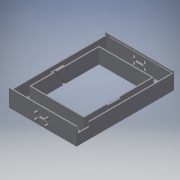
# Autodesk Inventor part: Frame V2.3
Saved by Autodesk Inventor 2018.3 (Build 223284000, 284)
## iProperties
Created: 2020-11-27
Part Number: Frame V2.3
Material: Generic
Document SubType Name: Modeling
Designer: daanv
Density: 1 g/cm^3
Appearance: Default
Author: daanv
Autodesk Inventor part; units mm, degrees
ref_plane "YZ Plane" through (0, 0, 0) normal (1, 0, 0) x (0, 1, 0)
ref_plane "XZ Plane" through (0, 0, 0) normal (0, 1, 0) x (-1, 0, 0)
ref_plane "XY Plane" through (0, 0, 0) normal (0, 0, 1) x (1, 0, 0)
sketch "Sketch1" plane through (0, 0, 0) normal (0, 0, 1) x (1, 0, 0)
  line L0 (0, 0) -> (90, 0)
  line L1 (90, 0) -> (90, 130)
  line L2 (90, 130) -> (0, 130)
  line L3 (0, 130) -> (0, 0)
  line L4 (10, 20) -> (80, 20)
  line L5 (80, 20) -> (80, 110)
  line L6 (80, 110) -> (10, 110)
  line L7 (10, 110) -> (10, 20)
  dimension "d0" = 90
  dimension "d1" = 130
  dimension "d2" = 70
  dimension "d3" = 90
  dimension "d16" = 20
  dimension "d17" = 20
  dimension "d18" = 10
  constraints: 16 end point, 4 parallel, 2 horizontal, 2 perpendicular
  measures "d0" distance of L2.end L1.end
  measures "d1" distance of L1.end L0.end
  measures "d2" distance of L6.end L5.end
  measures "d3" distance of L5.end L4.end
  measures "d16" distance between parallel lines of L2 L6
  measures "d17" distance between parallel lines of L0 L4
  measures "d18" distance between parallel lines of L1 L5
extrude "Extrusion1" add sketch "Sketch1" along normal blind 20
sketch "Sketch2" plane through (10, 20, 0) normal (1, 0, 0) x (0, 0, -1)
  line L0 (0, 90) -> (0, 0) projected
  line L1 (0, 42.1132) -> (-20, 30.5662)
  line L2 (-20, 110) -> (-20, -20) projected
  line L3 (0, 42.1132) -> (23.094, 42.1132) construction
  line L4 (-20, 30.5662) -> (-20, 33.6662)
  line L5 (-20, 33.6662) -> (0, 45.2132)
  line L6 (0, 42.1132) -> (0, 45.2132)
  point P0 (-20, 0)
  point P1 (0, -20)
  dimension "d6" = 210
  dimension "d7" = 3.1
  dimension "d8" = 26.4711
  constraints: 10 end point, 4 point on line, 1 collinear, 1 equal length, 1 horizontal, 1 parallel
  measures "d7" distance of L1.end L4.end
  measures "d8" distance from line of point (-20, 0) L1
extrude "Extrusion2" cut sketch "Sketch2" against normal blind 2.1
sketch "Sketch3" plane through (80, 20, 0) normal (-1, 0, 0) x (0, 0, 1)
  line L0 (0, 0) -> (0, 90) projected
  line L1 (20, 90) -> (20, 0) projected
  line L2 (0, 42.1132) -> (20, 30.5662)
  line L3 (0, 42.1132) -> (23.094, 42.1132) construction
  line L4 (20, 30.5662) -> (20, 33.6662)
  line L5 (20, 33.6662) -> (0, 45.2132)
  line L6 (0, 42.1132) -> (0, 45.2132)
  point P0 (0, -20)
  dimension "d11" = 30
  dimension "d12" = 3.1
  dimension "d13" = 26.4711
  constraints: 10 end point, 4 point on line, 1 equal length, 1 horizontal, 1 parallel
  measures "d11" angle of L2 L3
  measures "d12" distance of L2.end L4.end
  measures "d13" distance from line of L1.end L2
extrude "Extrusion3" cut sketch "Sketch3" against normal blind 2.1
sketch "Sketch4" plane through (0, 0, 0) normal (0, -1, 0) x (1, 0, 0)
  line L0 (0, 0) -> (90, 0) projected
  line L1 (90, 0) -> (90, 20) projected
  line L2 (0, 20) -> (90, 20) projected
  line L3 (0, 0) -> (0, 20) projected
  line L4 (55, 3) -> (35, 3)
  line L5 (35, 3) -> (35, 17)
  line L6 (35, 17) -> (55, 17)
  line L7 (55, 17) -> (55, 3)
  line L8 (53.2053, 7.41) -> (53.87, 5.3643)
  line L9 (53.87, 5.3643) -> (52.1298, 4.1)
  line L10 (52.1298, 4.1) -> (50.3897, 5.3643)
  line L11 (50.3897, 5.3643) -> (51.0543, 7.41)
  line L12 (51.0543, 7.41) -> (53.2053, 7.41)
  line L13 (38.9443, 7.41) -> (39.609, 5.3643)
  line L14 (39.609, 5.3643) -> (37.8689, 4.1)
  line L15 (37.8689, 4.1) -> (36.1287, 5.3643)
  line L16 (36.1287, 5.3643) -> (36.7934, 7.41)
  line L17 (36.7934, 7.41) -> (38.9443, 7.41)
  line L18 (38.9447, 15.55) -> (39.6093, 13.5043)
  line L19 (39.6093, 13.5043) -> (37.8692, 12.24)
  line L20 (37.8692, 12.24) -> (36.129, 13.5043)
  line L21 (36.129, 13.5043) -> (36.7937, 15.55)
  line L22 (36.7937, 15.55) -> (38.9447, 15.55)
  line L23 (53.2053, 15.55) -> (53.87, 13.5043)
  line L24 (53.87, 13.5043) -> (52.1298, 12.24)
  line L25 (52.1298, 12.24) -> (50.3897, 13.5043)
  line L26 (50.3897, 13.5043) -> (51.0543, 15.55)
  line L27 (51.0543, 15.55) -> (53.2053, 15.55)
  point P0 (52.1298, 5.9297)
  point P1 (37.8689, 5.9297)
  point P2 (37.8692, 14.0697)
  point P3 (52.1298, 14.0697)
  dimension "d19" = 20
  dimension "d20" = 14
  dimension "d21" = 3
  dimension "d22" = 3
  dimension "d23" = 35
  dimension "d24" = 35
  dimension "d25" = 1.45
  dimension "d26" = 1.45
  dimension "d27" = 1.1
  dimension "d28" = 1.1
  dimension "d29" = 12.11
  dimension "d30" = 1.13
  dimension "d31" = 1.13
  dimension "d32" = 4.83
  dimension "d33" = 4.83
  dimension "d34" = 1.129
  dimension "d35" = 1.1287
  constraints: 48 end point, 5 horizontal, 3 equal length, 2 parallel, 1 perpendicular, 44 other
  measures "d19" distance of L5.end L6.end
  measures "d20" distance of L4.end L5.end
  measures "d21" distance between parallel lines of L4 L0
  measures "d22" distance between parallel lines of L2 L6
  measures "d23" distance between parallel lines of L1 L7
  measures "d24" distance between parallel lines of L3 L5
  measures "d25" distance between parallel lines of L6 L27
  measures "d26" distance between parallel lines of L22 L6
  measures "d27" distance from line of L4 L9.end
  measures "d28" distance from line of L4 L14.end
  measures "d29" distance of L13.start L11.end
  measures "d30" distance from line of L7 L8.end
  measures "d31" distance from line of L7 L23.end
  measures "d32" distance from line of L12 L24.end
  measures "d33" distance from line of L17 L19.end
  measures "d34" distance from line of L5 L20.end
  measures "d35" distance from line of L5 L15.end
extrude "Extrusion4" add sketch "Sketch4" along normal blind 4 contours L8 L9 L10 L11 L12 | L13 L14 L15 L16 L17 | L18 L19 L20 L21 L22 | L23 L24 L25 L26 L27
chamfer "Chamfer1" distance 0.5 angle 45 20 edges at (52.1298, -4, 15.55) (50.722, -4, 14.5272) (51.2597, -4, 12.8722) (52.9999, -4, 12.8722) (53.5377, -4, 14.5272) (52.1298, -4, 7.41) (53.5377, -4, 6.3872) (52.9999, -4, 4.7322) (51.2597, -4, 4.7322) (50.722, -4, 6.3872) (39.277, -4, 14.5272) (38.7393, -4, 12.8722) (36.9991, -4, 12.8722) (36.4613, -4, 14.5272) (37.8692, -4, 15.55) (37.8689, -4, 7.41) (39.2767, -4, 6.3872) (38.7389, -4, 4.7322) (36.9988, -4, 4.7322) (36.461, -4, 6.3872)
sketch "Sketch5" plane through (0, 130, 0) normal (0, 1, 0) x (1, 0, 0)
  line L0 (90, 0) -> (0, 0) projected
  line L1 (0, 0) -> (0, -20) projected
  line L2 (90, -20) -> (0, -20) projected
  line L3 (90, 0) -> (90, -20) projected
  line L4 (55, -17) -> (35, -17)
  line L5 (35, -17) -> (35, -3)
  line L6 (35, -3) -> (55, -3)
  line L7 (55, -3) -> (55, -17)
  line L8 (51.9294, -7.9716) -> (49.9877, -6.5609)
  line L9 (49.9877, -6.5609) -> (50.7294, -4.2783)
  line L10 (50.7294, -4.2783) -> (53.1294, -4.2783)
  line L11 (53.1294, -4.2783) -> (53.871, -6.5609)
  line L12 (53.871, -6.5609) -> (51.9294, -7.9716)
  line L13 (52.13, -16.1116) -> (50.1884, -14.7009)
  line L14 (50.1884, -14.7009) -> (50.93, -12.4183)
  line L15 (50.93, -12.4183) -> (53.33, -12.4183)
  line L16 (53.33, -12.4183) -> (54.0716, -14.7009)
  line L17 (54.0716, -14.7009) -> (52.13, -16.1116)
  line L18 (37.84, -16.1116) -> (35.8984, -14.7009)
  line L19 (35.8984, -14.7009) -> (36.64, -12.4183)
  line L20 (36.64, -12.4183) -> (39.04, -12.4183)
  line L21 (39.04, -12.4183) -> (39.7816, -14.7009)
  line L22 (39.7816, -14.7009) -> (37.84, -16.1116)
  line L23 (37.6394, -7.9716) -> (35.6977, -6.5609)
  line L24 (35.6977, -6.5609) -> (36.4394, -4.2783)
  line L25 (36.4394, -4.2783) -> (38.8394, -4.2783)
  line L26 (38.8394, -4.2783) -> (39.581, -6.5609)
  line L27 (39.581, -6.5609) -> (37.6394, -7.9716)
  line L28 (50.5, -11.3) -> (39.5, -11.3)
  line L29 (39.5, -11.3) -> (39.5, -8.7)
  line L30 (39.5, -8.7) -> (50.5, -8.7)
  line L31 (50.5, -8.7) -> (50.5, -11.3)
  point P0 (51.9294, -5.93)
  point P1 (52.13, -14.07)
  point P2 (37.84, -14.07)
  point P3 (37.6394, -5.93)
  dimension "d41" = 20
  dimension "d42" = 14
  dimension "d43" = 3
  dimension "d44" = 3
  dimension "d45" = 35
  dimension "d46" = 35
  dimension "d142" = 2.4
  dimension "d144" = 2.4
  dimension "d148" = 2.4
  dimension "d151" = 4.4468
  dimension "d154" = 2.4
  dimension "d158" = 11.89
  dimension "d159" = 11
  dimension "d160" = 2.6
  dimension "d161" = 4.5
  dimension "d162" = 5.7
  dimension "d164" = 2.87
  dimension "d165" = 2.93
  dimension "d168" = 14.29
  dimension "d170" = 8.14
  dimension "d172" = 2.93
  dimension "d173" = 8.14
  dimension "d174" = 4.4468
  dimension "d175" = 0.6977
  dimension "d176" = 1.129
  dimension "d177" = 14.29
  constraints: 56 end point, 5 horizontal, 4 parallel, 2 perpendicular, 44 other
  measures "d41" distance of L5.end L6.end
  measures "d42" distance of L4.end L5.end
  measures "d43" distance between parallel lines of L2 L4
  measures "d44" distance between parallel lines of L0 L6
  measures "d45" distance between parallel lines of L3 L7
  measures "d46" distance between parallel lines of L1 L5
  measures "d142" distance of L9.end L10.end
  measures "d144" distance of L14.end L15.end
  measures "d148" distance of L19.end L20.end
  measures "d151" distance from line of L8.start L15
  measures "d154" distance of L24.end L25.end
  measures "d158" distance of L25.end L9.end
  measures "d159" distance of L29.end L30.end
  measures "d160" distance of L28.end L29.end
  measures "d161" distance between parallel lines of L7 L31
  measures "d162" distance between parallel lines of L6 L30
  measures "d164" distance from line of point (52.13, -14.07) L7
  measures "d165" distance from line of L4 point (37.84, -14.07)
  measures "d168" distance of point (37.639, -5.93) point (51.929, -5.93)
  measures "d170" vertical distance of point (37.639, -5.93) point (37.84, -14.07)
  measures "d172" distance from line of L4 point (52.13, -14.07)
  measures "d173" vertical distance of point (52.13, -14.07) point (51.929, -5.93)
  measures "d174" distance from line of L20 L23.start
  measures "d175" distance from line of L5 L23.end
  measures "d176" distance from line of L7 L11.end
  measures "d177" distance of point (37.84, -14.07) point (52.13, -14.07)
extrude "Extrusion5" cut sketch "Sketch5" against normal blind 4 contours L8 L9 L10 L11 L12 | L13 L14 L15 L16 L17 | L18 L19 L20 L21 L22 | L23 L24 L25 L26 L27 | L28 L29 L30 L31
chamfer "Chamfer2" distance 0.5 angle 45 20 edges at (51.1592, 130, 15.4062) (53.1008, 130, 15.4062) (53.7008, 130, 13.5596) (52.13, 130, 12.4183) (50.5592, 130, 13.5596) (50.9586, 130, 7.2662) (52.9002, 130, 7.2662) (53.5002, 130, 5.4196) (51.9294, 130, 4.2783) (50.3586, 130, 5.4196) (39.4108, 130, 13.5596) (38.8108, 130, 15.4062) (36.8692, 130, 15.4062) (36.2692, 130, 13.5596) (37.84, 130, 12.4183) (36.6686, 130, 7.2662) (38.6102, 130, 7.2662) (39.2102, 130, 5.4196) (37.6394, 130, 4.2783) (36.0686, 130, 5.4196)
sketch "Sketch6" plane through (0, 0, 20) normal (0, 0, 1) x (1, 0, 0)
  line L0 (0, 0) -> (90, 0) projected
  line L1 (90, 0) -> (90, 130) projected
  line L2 (90, 130) -> (0, 130) projected
  line L3 (1.5, 130) -> (1.5, 1.5)
  line L4 (0, 0) -> (90, 0) projected
  line L5 (1.5, 1.5) -> (88.5, 1.5)
  line L6 (88.5, 1.5) -> (88.5, 128.5)
  line L7 (88.5, 128.5) -> (1.5, 128.5)
  line L8 (8.5, 111.5) -> (8.5, 65.5)
  line L9 (10, 65.2132) -> (7.9, 65.2132) projected
  line L10 (8.5, 65.5) -> (6.5, 65.5)
  line L11 (6.5, 65.5) -> (6.5, 49.066)
  line L12 (6.5, 49.066) -> (8.5, 49.066)
  line L13 (8.5, 49.066) -> (8.5, 18.5)
  line L14 (8.5, 18.5) -> (81.5, 18.5)
  line L15 (81.5, 18.5) -> (81.5, 49.066)
  line L16 (81.5, 49.066) -> (83.5, 49.066)
  line L17 (83.5, 49.066) -> (83.5, 65.5)
  line L18 (83.5, 65.5) -> (81.5, 65.5)
  line L19 (81.5, 65.5) -> (81.5, 111.5)
  line L20 (81.5, 111.5) -> (8.5, 111.5)
  dimension "d79" = 128.5
  dimension "d80" = 87
  dimension "d81" = 127
  dimension "d82" = 46
  dimension "d83" = 2
  dimension "d84" = 16.434
  dimension "d85" = 2
  dimension "d86" = 30.566
  dimension "d87" = 73
  dimension "d88" = 2
  constraints: 32 end point, 10 perpendicular, 6 point on line, 2 parallel, 1 horizontal
  measures "d79" distance of L3.start L3.end
  measures "d80" distance of L3.end L5.end
  measures "d81" distance of L5.end L6.end
  measures "d82" distance of L8.start L8.end
  measures "d83" distance of L8.end L10.end
  measures "d84" distance of L10.end L11.end
  measures "d85" distance of L11.end L12.end
  measures "d86" distance of L12.end L13.end
  measures "d87" distance of L13.end L14.end
  measures "d88" distance of L15.end L16.end
extrude "Extrusion6" cut sketch "Sketch6" against normal blind 18
sketch "Sketch7" plane through (0, 0, 0) normal (0, -1, 0) x (1, 0, 0)
  line L0 (0, 0) -> (90, 0) projected
  line L1 (90, 0) -> (90, 20) projected
  line L2 (0, 20) -> (90, 20) projected
  line L3 (0, 0) -> (0, 20) projected
  line L4 (39.5, 8.7) -> (50.5, 8.7)
  line L5 (50.5, 8.7) -> (50.5, 11.3)
  line L6 (50.5, 11.3) -> (39.5, 11.3)
  line L7 (39.5, 11.3) -> (39.5, 8.7)
  dimension "d100" = 11
  dimension "d101" = 2.6
  dimension "d102" = 8.7
  dimension "d103" = 39.5
  dimension "d104" = 39.5
  dimension "d105" = 8.7
  constraints: 8 end point, 2 parallel, 1 horizontal, 1 perpendicular
  measures "d100" distance of L4.start L4.end
  measures "d101" distance of L4.end L5.end
  measures "d102" distance between parallel lines of L2 L6
  measures "d103" distance between parallel lines of L3 L7
  measures "d104" distance between parallel lines of L1 L5
  measures "d105" distance between parallel lines of L0 L4
extrude "Extrusion7" cut sketch "Sketch7" against normal blind 10 contours L7 L6 L5 L4
sketch "Sketch16" plane through (90, 0, 0) normal (1, 0, 0) x (0, 0, -1)
  line L0 (0, 0) -> (0, 130) projected
  line L1 (0, 0) -> (-20, 0) projected
  line L2 (-20, 1.5) -> (-20, 128.5) projected
  line L3 (-20, 2) -> (-14.283, 2)
  line L4 (-14.283, 2) -> (-14.283, 17)
  line L5 (-14.283, 17) -> (-20, 17)
  line L6 (-20, 17) -> (-20, 2)
  dimension "d178" = 2
  dimension "d179" = 15
  dimension "d180" = 14.283
  constraints: 8 end point, 2 parallel, 1 horizontal, 1 perpendicular, 1 point on line
  measures "d178" distance between parallel lines of L1 L3
  measures "d179" distance of L3.end L4.end
  measures "d180" distance between parallel lines of L0 L4
extrude "Extrusion15" cut sketch "Sketch16" against normal blind 10
sketch "Sketch17" plane through (0, 0, 20) normal (0, 0, 1) x (1, 0, 0)
  line L0 (88.5, 1.5) -> (1.5, 1.5) projected
  line L1 (1.5, 128.5) -> (88.5, 128.5) projected
  line L2 (90, 17) -> (90, 130) projected
  line L3 (0, 0) -> (90, 0) projected
  line L4 (90, 0) -> (90, 2) projected
  line L5 (0, 0) -> (90, 0)
  line L6 (90, 0) -> (90, 1.5)
  line L7 (90, 1.5) -> (0, 1.5)
  line L8 (0, 1.5) -> (0, 0)
  line L9 (0, 130) -> (90, 130)
  line L10 (90, 130) -> (90, 128.5)
  line L11 (90, 128.5) -> (0, 128.5)
  line L12 (0, 128.5) -> (0, 130)
  constraints: 16 end point, 4 parallel, 4 point on line, 2 horizontal, 2 perpendicular
extrude "Extrusion16" add sketch "Sketch17" along normal blind 2.8
sketch "Sketch18" plane through (90, 0, 0) normal (1, 0, 0) x (0, 0, -1)
  line L0 (-20, 1.5) -> (-20, 2) projected
  line L1 (-22.8, 0) -> (-22.8, 1.5) projected
  line L2 (-22.8, 128.5) -> (-22.8, 130) projected
  line L3 (-20, 128.5) -> (-22.8, 128.5) projected
  line L4 (-20, 1.5) -> (-22.8, 1.5) projected
  line L5 (-21.55, 1.5) -> (-20.05, 1.5)
  line L6 (-20.05, 1.5) -> (-20.05, 0.7)
  line L7 (-20.05, 0.7) -> (-21.55, 0.7)
  line L8 (-21.55, 0.7) -> (-21.55, 1.5)
  line L9 (-21.55, 128.5) -> (-20.05, 128.5)
  line L10 (-20.05, 128.5) -> (-20.05, 129.3)
  line L11 (-20.05, 129.3) -> (-21.55, 129.3)
  line L12 (-21.55, 129.3) -> (-21.55, 128.5)
  dimension "d185" = 1.5
  dimension "d186" = 0.8
  dimension "d187" = 1.25
  dimension "d188" = 0.05
  dimension "d189" = 1.5
  dimension "d190" = 0.8
  dimension "d191" = 1.25
  constraints: 16 end point, 4 parallel, 2 horizontal, 2 perpendicular, 2 point on line
  measures "d185" distance of L6.end L7.end
  measures "d186" distance of L5.end L6.end
  measures "d187" distance between parallel lines of L1 L8
  measures "d188" distance between parallel lines of L0 L6
  measures "d189" distance of L11.end L10.end
  measures "d190" distance of L10.end L9.end
  measures "d191" distance between parallel lines of L2 L12
extrude "Extrusion17" cut sketch "Sketch18" against normal blind 85
body "Solid1"
